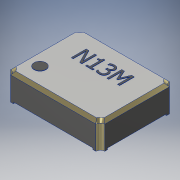
# Autodesk Inventor part: Crystal_TXO-3225
Saved by Autodesk Inventor 2018 (Build 220112000, 112)
## iProperties
Created: 2016-08-15
Part Number: Crystal_TXO-3225
Material: Aluminum 6061
Document SubType Name: Modeling
Designer: Bradley
Density: 2.7 g/cm^3
Appearance: Aluminum - Flat
Author: Bradley
Autodesk Inventor part; units mm, degrees
ref_plane "YZ Plane" through (0, 0, 0) normal (1, 0, 0) x (0, 1, 0)
ref_plane "XZ Plane" through (0, 0, 0) normal (0, 1, 0) x (-1, 0, 0)
ref_plane "XY Plane" through (0, 0, 0) normal (0, 0, 1) x (1, 0, 0)
sketch "Sketch1" plane through (0, 0, 0) normal (0, 1, 0) x (-1, 0, 0)
  line L0 (-1.6, 1.25) -> (1.6, 1.25)
  line L1 (1.6, 1.25) -> (1.6, -1.25)
  line L2 (1.6, -1.25) -> (-1.6, -1.25)
  line L3 (-1.6, -1.25) -> (-1.6, 1.25)
  line L4 (-1.6, 1.25) -> (1.6, -1.25) construction
  line L5 (1.6, 1.25) -> (-1.6, -1.25) construction
  arc A0 (1.6, -1.1) -> (1.45, -1.25) centre (1.6, -1.25) ccw
  arc A1 (-1.45, -1.25) -> (-1.6, -1.1) centre (-1.6, -1.25) ccw
  arc A2 (-1.6, 1.1) -> (-1.45, 1.25) centre (-1.6, 1.25) ccw
  arc A3 (1.45, 1.25) -> (1.6, 1.1) centre (1.6, 1.25) ccw
  point P0 (0, 0)
  dimension "d0" = 3.2
  dimension "d1" = 2.5
  dimension "d4" = 0.15
  constraints: 12 end point, 8 point on circle, 8 point on line, 4 centre point, 4 coincident, 3 equal radius, 2 midpoint, 2 parallel, 1 horizontal, 1 perpendicular
  measures "d0" distance of L1.end L2.end
  measures "d1" distance of L0.end L1.end
  measures "d4" radius of A0
extrude "Extrusion1" add sketch "Sketch1" along normal mid plane 0.85 contours L0 A3 L1 A0 L2 A1 L3 A2
chamfer "Chamfer1" distance 0.1 angle 45 8 edges at (0, 0.425, 1.25) (-1.4939, 0.425, 1.1439) (-1.6, 0.425, 0) (-1.4939, 0.425, -1.1439) (0, 0.425, -1.25) (1.4939, 0.425, -1.1439) (1.6, 0.425, 0) (1.4939, 0.425, 1.1439)
sketch "Sketch3" plane through (0, 0.425, 0) normal (0, 1, 0) x (1, 0, 0)
  line L0 (-1.3709, 1.15) -> (1.3709, 1.15) projected
  arc A0 (-1.5, 1.0209) -> (-1.3709, 1.15) centre (-1.6, 1.25) ccw projected
  line L1 (-1.5, -1.0209) -> (-1.5, 1.0209) projected
  arc A1 (-1.3709, -1.15) -> (-1.5, -1.0209) centre (-1.6, -1.25) ccw projected
  line L2 (1.3709, -1.15) -> (-1.3709, -1.15) projected
  arc A2 (1.5, -1.0209) -> (1.3709, -1.15) centre (1.6, -1.25) ccw projected
  line L3 (1.5, 1.0209) -> (1.5, -1.0209) projected
  arc A3 (1.3709, 1.15) -> (1.5, 1.0209) centre (1.6, 1.25) ccw projected
  line L4 (1.5, 1.0209) -> (1.5, -1.0209) construction
  line L5 (1.5, 0.1868) -> (-1.5, 0.1868) construction
  circle A4 centre (-1.1, -0.6) radius 0.2
  line L6 (-0.4613, 0.1868) -> (-0.5359, 0.1868)
  line L7 (-0.5359, 0.1868) -> (-0.7571, 0.6179)
  line L8 (-0.7571, 0.6179) -> (-0.7571, 0.1868)
  line L9 (-0.7571, 0.1868) -> (-0.8191, 0.1868)
  line L10 (-0.8191, 0.1868) -> (-0.8191, 0.6868)
  line L11 (-0.8191, 0.6868) -> (-0.7247, 0.6868)
  line L12 (-0.7247, 0.6868) -> (-0.5233, 0.2909)
  line L13 (-0.5233, 0.2909) -> (-0.5233, 0.6868)
  line L14 (-0.5233, 0.6868) -> (-0.4613, 0.6868)
  line L15 (-0.4613, 0.6868) -> (-0.4613, 0.1868)
  line L16 (-0.091, 0.1868) -> (-0.3349, 0.1868)
  line L17 (-0.3349, 0.1868) -> (-0.3349, 0.2378)
  line L18 (-0.3349, 0.2378) -> (-0.2441, 0.2378)
  line L19 (-0.2441, 0.2378) -> (-0.2441, 0.5729)
  line L20 (-0.2441, 0.5729) -> (-0.3349, 0.5729)
  line L21 (-0.3349, 0.5729) -> (-0.3349, 0.6187)
  spline S0 degree 2 poles (-0.3349, 0.6187) (-0.2834, 0.6187) (-0.2348, 0.6479) (-0.2316, 0.6884) knots 0 0 0 1 2 2 2
  line L22 (-0.2316, 0.6884) -> (-0.1797, 0.6884)
  line L23 (-0.1797, 0.6884) -> (-0.1797, 0.2378)
  line L24 (-0.1797, 0.2378) -> (-0.091, 0.2378)
  line L25 (-0.091, 0.2378) -> (-0.091, 0.1868)
  spline S1 degree 2 poles (0.1359, 0.6393) (0.1177, 0.6393) (0.0816, 0.6304) (0.0642, 0.6235) knots 0 0 0 1 2 2 2
  spline S2 degree 2 poles (0.0642, 0.6235) (0.048, 0.6167) (0.0241, 0.6021) (0.0148, 0.5956) knots 0 0 0 1 2 2 2
  line L26 (0.0148, 0.5956) -> (0.0107, 0.5956)
  line L27 (0.0107, 0.5956) -> (0.0107, 0.6665)
  spline S3 degree 2 poles (0.0107, 0.6665) (0.0326, 0.6782) (0.1076, 0.6973) (0.1412, 0.6973) knots 0 0 0 1 2 2 2
  spline S4 degree 2 poles (0.1412, 0.6973) (0.1752, 0.6973) (0.2259, 0.6835) (0.2466, 0.6689) knots 0 0 0 1 2 2 2
  spline S5 degree 2 poles (0.2466, 0.6689) (0.2684, 0.6531) (0.2911, 0.6073) (0.2911, 0.5765) knots 0 0 0 1 2 2 2
  spline S6 degree 2 poles (0.2911, 0.5765) (0.2911, 0.5352) (0.2368, 0.4728) (0.1987, 0.4647) knots 0 0 0 1 2 2 2
  line L28 (0.1987, 0.4647) -> (0.1987, 0.4599)
  spline S7 degree 2 poles (0.1987, 0.4599) (0.2145, 0.4566) (0.2506, 0.442) (0.266, 0.4274) knots 0 0 0 1 2 2 2
  spline S8 degree 2 poles (0.266, 0.4274) (0.2814, 0.4133) (0.3009, 0.3679) (0.3009, 0.3351) knots 0 0 0 1 2 2 2
  spline S9 degree 2 poles (0.3009, 0.3351) (0.3009, 0.3014) (0.2778, 0.2443) (0.2567, 0.2224) knots 0 0 0 1 2 2 2
  spline S10 degree 2 poles (0.2567, 0.2224) (0.2348, 0.1997) (0.1728, 0.1762) (0.1335, 0.1762) knots 0 0 0 1 2 2 2
  spline S11 degree 2 poles (0.1335, 0.1762) (0.0958, 0.1762) (0.0221, 0.1945) (-0.003, 0.207) knots 0 0 0 1 2 2 2
  line L29 (-0.003, 0.207) -> (-0.003, 0.2779)
  line L30 (-0.003, 0.2779) -> (0.0018, 0.2779)
  spline S12 degree 2 poles (0.0018, 0.2779) (0.0229, 0.2625) (0.0942, 0.2342) (0.1295, 0.2342) knots 0 0 0 1 2 2 2
  spline S13 degree 2 poles (0.1295, 0.2342) (0.1501, 0.2342) (0.1915, 0.2471) (0.2052, 0.2621) knots 0 0 0 1 2 2 2
  spline S14 degree 2 poles (0.2052, 0.2621) (0.2186, 0.2771) (0.2328, 0.3128) (0.2328, 0.3399) knots 0 0 0 1 2 2 2
  spline S15 degree 2 poles (0.2328, 0.3399) (0.2328, 0.3671) (0.217, 0.4023) (0.2028, 0.4124) knots 0 0 0 1 2 2 2
  spline S16 degree 2 poles (0.2028, 0.4124) (0.1886, 0.4226) (0.1501, 0.4303) (0.1274, 0.4303) knots 0 0 0 1 2 2 2
  line L31 (0.1274, 0.4303) -> (0.0991, 0.4303)
  line L32 (0.0991, 0.4303) -> (0.0991, 0.4858)
  line L33 (0.0991, 0.4858) -> (0.1214, 0.4858)
  spline S17 degree 2 poles (0.1214, 0.4858) (0.1663, 0.4858) (0.2231, 0.5287) (0.2231, 0.5697) knots 0 0 0 1 2 2 2
  spline S18 degree 2 poles (0.2231, 0.5697) (0.2231, 0.5887) (0.2085, 0.6158) (0.1967, 0.624) knots 0 0 0 1 2 2 2
  spline S19 degree 2 poles (0.1967, 0.624) (0.1842, 0.6325) (0.1534, 0.6393) (0.1359, 0.6393) knots 0 0 0 1 2 2 2
  line L34 (0.8191, 0.1868) -> (0.7526, 0.1868)
  line L35 (0.7526, 0.1868) -> (0.7526, 0.6175)
  line L36 (0.7526, 0.6175) -> (0.6222, 0.3245)
  line L37 (0.6222, 0.3245) -> (0.5816, 0.3245)
  line L38 (0.5816, 0.3245) -> (0.4524, 0.6175)
  line L39 (0.4524, 0.6175) -> (0.4524, 0.1868)
  line L40 (0.4524, 0.1868) -> (0.3904, 0.1868)
  line L41 (0.3904, 0.1868) -> (0.3904, 0.6868)
  line L42 (0.3904, 0.6868) -> (0.4812, 0.6868)
  line L43 (0.4812, 0.6868) -> (0.606, 0.4084)
  line L44 (0.606, 0.4084) -> (0.7267, 0.6868)
  line L45 (0.7267, 0.6868) -> (0.8191, 0.6868)
  line L46 (0.8191, 0.6868) -> (0.8191, 0.1868)
  point P0 (0, 0)
  dimension "d27" = 0.4
  dimension "d28" = 0.6
  dimension "d29" = 1.1
  constraints: 2 end point, 2 point on line, 1 centre point, 1 horizontal, 1 perpendicular
  measures "d27" diameter of A4
  measures "d28" vertical distance of point (0, 0) A4.centre
  measures "d29" horizontal distance of point (0, 0) A4.centre
extrude "Extrusion3" add sketch "Sketch3" along normal blind 0.01 contours A4 | L6 L7 L8 L9 L10 L11 L12 L13 L14 L15 | L16 L17 L18 L19 L20 L21 S0 L22 L23 L24 L25 | S1 S2 L26 L27 S3 S4 S5 S6 L28 S7 S8 S9 S10 S11 L29 L30 S12 S13 S14 S15 S16 L31 L32 L33 S17 S18 S19 | L34 L35 L36 L37 L38 L39 L40 L41 L42 L43 L44 L45 L46
sketch "Sketch4" plane through (0, -0.425, 0) normal (0, -1, 0) x (1, 0, 0)
  line L0 (-1.6, 1.1) -> (-1.6, -1.1) projected
  arc A0 (-1.45, -1.25) -> (-1.6, -1.1) centre (-1.6, -1.25) ccw projected
  line L1 (-1.45, -1.25) -> (1.45, -1.25) projected
  arc A1 (1.6, -1.1) -> (1.45, -1.25) centre (1.6, -1.25) ccw projected
  line L2 (1.6, -1.1) -> (1.6, 1.1) projected
  arc A2 (1.45, 1.25) -> (1.6, 1.1) centre (1.6, 1.25) ccw projected
  line L3 (1.45, 1.25) -> (-1.45, 1.25) projected
  arc A3 (-1.6, 1.1) -> (-1.45, 1.25) centre (-1.6, 1.25) ccw projected
  line L4 (1.35, 1.25) -> (1.35, 1.19)
  line L5 (1.35, 1.19) -> (0.94, 1.19)
  line L6 (0.94, 1.19) -> (0.94, 0.35)
  line L7 (0.94, 0.35) -> (1.54, 0.35)
  line L8 (1.54, 0.35) -> (1.54, 1)
  line L9 (1.54, 1) -> (1.6, 1)
  line L10 (-1.6, -1.1) -> (-1.6, 1.1) projected
  line L11 (-1.6, 1) -> (-1.54, 1)
  line L12 (-1.54, 1) -> (-1.54, 0.35)
  line L13 (-1.54, 0.35) -> (-0.94, 0.35)
  line L14 (-0.94, 0.35) -> (-0.94, 1.19)
  line L15 (-0.94, 1.19) -> (-1.35, 1.19)
  line L16 (-1.35, 1.19) -> (-1.35, 1.25)
  line L17 (1.45, -1.25) -> (-1.45, -1.25) projected
  line L18 (-1.35, -1.25) -> (-1.35, -1.19)
  line L19 (-1.35, -1.19) -> (-0.94, -1.19)
  line L20 (-0.94, -1.19) -> (-0.94, -0.35)
  line L21 (-0.94, -0.35) -> (-1.54, -0.35)
  line L22 (-1.54, -0.35) -> (-1.54, -1)
  line L23 (-1.54, -1) -> (-1.6, -1)
  line L24 (1.6, -1) -> (1.54, -1)
  line L25 (1.54, -1) -> (1.54, -0.35)
  line L26 (1.54, -0.35) -> (0.94, -0.35)
  line L27 (0.94, -0.35) -> (0.94, -1.19)
  line L28 (0.94, -1.19) -> (1.35, -1.19)
  line L29 (1.35, -1.19) -> (1.35, -1.25)
  point P0 (0, 0)
  dimension "d20" = 0.84
  dimension "d21" = 0.6
  dimension "d22" = 1.88
  dimension "d23" = 0.25
  dimension "d24" = 0.25
  constraints: 48 end point, 20 point on line, 15 perpendicular, 7 equal length, 6 collinear, 1 horizontal, 1 parallel, 1 vertical
  measures "d20" distance of L5.end L6.end
  measures "d21" distance of L6.end L7.end
  measures "d22" distance between parallel lines of L14 L6
  measures "d23" distance between parallel lines of L4 L2
  measures "d24" distance between parallel lines of L9 L3
extrude "Extrusion5" add sketch "Sketch4" along normal blind 0.05 contours A3 L3 L16 L15 L14 L13 L12 L11 L0 | L23 L22 L21 L20 L19 L18 L1 A0 L0 | L3 A2 L2 L9 L8 L7 L6 L5 L4 | L29 L28 L27 L26 L25 L24 L2 A1 L1
equation "\"d24\" = d23"
body "Solid1"
